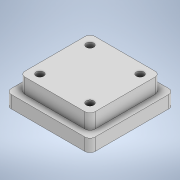
# Autodesk Inventor part: Деталь2
Saved by Autodesk Inventor 2020.2 (Build 242310000, 310)
## iProperties
Created: 2026-03-04
Part Number: Деталь2
Material: Типовые
Document SubType Name: Modeling
Designer: tankfpv
Density: 1 g/cm^3
Appearance: По умолчанию
Author: tankfpv
Autodesk Inventor part; units mm, degrees
ref_plane "YZ Plane" through (0, 0, 0) normal (1, 0, 0) x (0, 1, 0)
ref_plane "XZ Plane" through (0, 0, 0) normal (0, 1, 0) x (-1, 0, 0)
ref_plane "XY Plane" through (0, 0, 0) normal (0, 0, 1) x (1, 0, 0)
sketch "Эскиз1" plane through (0, 0, 0) normal (0, 1, 0) x (-1, 0, 0)
  line L0 (-14.75, 16.75) -> (14.75, 16.75)
  line L1 (16.75, 14.75) -> (16.75, -14.75)
  line L2 (14.75, -16.75) -> (-14.75, -16.75)
  line L3 (-16.75, -14.75) -> (-16.75, 14.75)
  line L4 (-16.75, 16.75) -> (16.75, -16.75) construction
  line L5 (16.75, 16.75) -> (-16.75, -16.75) construction
  arc A0 (16.75, 14.75) -> (14.75, 16.75) centre (14.75, 14.75) ccw
  arc A1 (14.75, -16.75) -> (16.75, -14.75) centre (14.75, -14.75) ccw
  arc A2 (-16.75, -14.75) -> (-14.75, -16.75) centre (-14.75, -14.75) ccw
  arc A3 (-14.75, 16.75) -> (-16.75, 14.75) centre (-14.75, 14.75) ccw
  point P0 (0, 0)
  dimension "d0" = 33.5
  dimension "d1" = 33.5
  dimension "d2" = 2
  constraints: 12 end point, 8 point on circle, 8 point on line, 8 tangent, 4 centre point, 3 equal radius, 2 midpoint, 2 parallel, 1 horizontal, 1 perpendicular
  measures "d0" distance of L4.end L5.end
  measures "d1" distance of L5.start L4.end
  measures "d2" radius of A0
extrude "Выдавливание1" add sketch "Эскиз1" along normal blind 5
sketch "Эскиз2" plane through (0, 5, 0) normal (0, 1, 0) x (1, 0, 0)
  line L0 (12, 14) -> (-12, 14)
  line L1 (-14, 12) -> (-14, -12)
  line L2 (-12, -14) -> (12, -14)
  line L3 (14, -12) -> (14, 12)
  line L4 (14, 14) -> (-14, -14) construction
  line L5 (-14, 14) -> (14, -14) construction
  line L6 (10, -10) -> (-10, -10)
  line L7 (-10, -10) -> (-10, 10)
  line L8 (-10, 10) -> (10, 10)
  line L9 (10, 10) -> (10, -10)
  line L10 (10, -10) -> (-10, 10) construction
  line L11 (-10, -10) -> (10, 10) construction
  circle A0 centre (-10, -10) radius 1.5
  circle A1 centre (-10, 10) radius 1.5
  circle A2 centre (10, 10) radius 1.5
  circle A3 centre (10, -10) radius 1.5
  arc A4 (-14, -12) -> (-12, -14) centre (-12, -12) ccw
  arc A5 (12, -14) -> (14, -12) centre (12, -12) ccw
  arc A6 (14, 12) -> (12, 14) centre (12, 12) ccw
  arc A7 (-12, 14) -> (-14, 12) centre (-12, 12) ccw
  point P0 (0, 0)
  dimension "d5" = 28
  dimension "d6" = 28
  dimension "d7" = 20
  dimension "d8" = 20
  dimension "d9" = 3
  dimension "d10" = 3
  dimension "d11" = 3
  dimension "d12" = 3
  dimension "d13" = 2
  constraints: 24 end point, 8 centre point, 8 point on circle, 8 point on line, 8 tangent, 4 coincident, 4 midpoint, 4 parallel, 3 equal radius, 2 horizontal, 2 perpendicular
  measures "d5" distance of L5.end L4.end
  measures "d6" distance of L4.end L5.start
  measures "d7" distance of L7.end L8.end
  measures "d8" distance of L6.end L7.end
  measures "d9" diameter of A0
  measures "d10" diameter of A1
  measures "d11" diameter of A2
  measures "d12" diameter of A3
  measures "d13" radius of A4
extrude "Выдавливание2" add sketch "Эскиз2" along normal blind 6 separate body contours A6 L3 A5 L2 A4 L1 A7 L0 | A0 L7 A1 L8 A2 L9 A3 L6
sketch "Эскиз3" plane through (0, 11, 0) normal (0, 1, 0) x (1, 0, 0)
  arc A0 (-12, 14) -> (-14, 12) centre (-12, 12) ccw projected
  line L0 (-14, 12) -> (-14, -12) projected
  arc A1 (-14, -12) -> (-12, -14) centre (-12, -12) ccw projected
  line L1 (-12, -14) -> (12, -14) projected
  arc A2 (12, -14) -> (14, -12) centre (12, -12) ccw projected
  line L2 (14, -12) -> (14, 12) projected
  arc A3 (14, 12) -> (12, 14) centre (12, 12) ccw projected
  line L3 (12, 14) -> (-12, 14) projected
  circle A4 centre (10, 10) radius 1.5 projected
  circle A5 centre (-10, 10) radius 1.5 projected
  circle A6 centre (-10, -10) radius 1.5 projected
  circle A7 centre (10, -10) radius 1.5 projected
  point P0 (0, 0)
extrude "Выдавливание3" cut sketch "Эскиз3" against normal blind 20 contours A4 | A5 | A6 | A7 bodies 1
